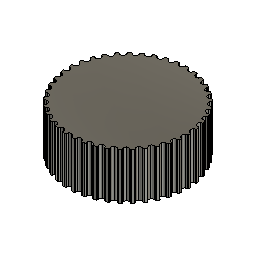
gear_41z (Autodesk Fusion 360 design; units mm, degrees)
Autodesk Fusion 360 part; units mm, degrees
sketch "Sketch1" plane through (0, 0, 0) normal (0, 0, 1) x (1, 0, 0) in component "gt2 pulley"
  circle A0 centre (0, 0) radius 13.0507 construction
  circle A1 centre (0, 0) radius 12.0467 construction
  line L0 (0, 0) -> (0, 13.0507) construction
  line L1 (0, 0) -> (0.999, 13.0124) construction
  line L2 (0, 0) -> (1.4084, 12.9745) construction
  circle A2 centre (0, 0) radius 12.7967 construction
  arc A3 (0.3832, 12.6546) -> (0.4455, 12.3686) centre (1.3809, 12.722) ccw
  circle A4 centre (0, 0) radius 12.6467 construction
  arc A5 (0.2363, 12.7945) -> (0, 12.7967) centre (0, 0) ccw
  arc A6 (0.3832, 12.6546) -> (0.2363, 12.7945) centre (0.2336, 12.6445) ccw
  arc A7 (0.4455, 12.3686) -> (0.9222, 12.0114) centre (0.9647, 12.5647) ccw
  arc A8 (0, 12.7967) -> (-0.2363, 12.7945) centre (0, 0) ccw
  arc A9 (-0.2363, 12.7945) -> (-0.3832, 12.6546) centre (-0.2336, 12.6445) ccw
  arc A10 (-0.4455, 12.3686) -> (-0.3832, 12.6546) centre (-1.3809, 12.722) ccw
  arc A11 (-0.9223, 12.0113) -> (-0.4455, 12.3686) centre (-0.9647, 12.5647) ccw
  arc A12 (0.9222, 12.0114) -> (-0.9222, 12.0114) centre (0, 0) ccw
  point P0 (1.3809, 12.722)
  point P1 (0, 12.7967)
  dimension "d18" = 26.1014
  dimension "d19" = 4.39
  dimension "d22" = 1.004
  dimension "d24" = 0.75
  dimension "d26" = 1
  dimension "d27" = 0.15
  dimension "d28" = 0.15
  dimension "d47" = 0.555
  dimension "d52" = 3.812
  constraint coincident A0.centre A1.centre
  constraint coincident A0 L0.end
  constraint vertical L0
  constraint coincident A0 L1.end
  constraint coincident A0 L2.end
  constraint concentric A1 A2
  constraint coincident A1 A7.end
  constraint coincident L1 A7.end
  constraint coincident A2 P0
  constraint coincident L2 P0
  constraint coincident P0 A3.centre
  constraint coincident A2 P1
  constraint coincident L0 P1
  constraint concentric A2 A4
  constraint coincident P1 A5.end
  constraint coincident A4 A6.centre
  constraint coincident A3.start A6.start
  constraint tangent A3 A6
  constraint tangent A3 A7
  constraint symmetric L0 A7.end A12.end
  constraint symmetric L0 A3.start A9.end
  constraint symmetric L0 A3.end A10.start
  constraint symmetric L0 A3 A10
  constraint symmetric L0 A5.start A8.end
  constraint symmetric L0 P1 A5.end
  constraint symmetric L0 A5 A8
  constraint symmetric L0 A6 A9
  constraint symmetric L0 A7 A11
  constraint coincident A1 A11.start
  constraint tangent A1 A7
  constraint coincident L1 A7.centre
  measures "d18" diameter of A0
  measures "d19" angle of L0 L1
  measures "d22" distance of A0 A1
  measures "d24" distance of A1 A2
  measures "d26" radius of A3
  measures "d27" distance of A2 A4
  measures "d28" radius of A6
  measures "d47" radius of A7
extrude "Extrude1" add sketch "Sketch1" along normal blind 10 makes body 1
pattern_circular "C-Pattern1" count 41 over 360 about axis through (0, 0, 1.75) along (0, 0, 1) of bodies 1 makes body 2 at (-2.5449, 11.7748, 6.6667) makes body 3 at (-4.3125, 11.2483, 6.6667) makes body 4 at (-4.6929, 11.095, 3.3333) makes body 5 at (-7.5054, 9.423, 6.6667) makes body 6 at (-7.8218, 9.162, 3.3333) makes body 7 at (-9.1287, 7.8607, 3.3333) makes body 8 at (-10.2216, 6.3751, 3.3333) makes body 9 at (-11.5601, 3.3893, 6.6667) makes body 10 at (-11.6688, 2.9939, 3.3333) makes body 11 at (-12.044, -0.2565, 6.6667) makes body 12 at (-11.8637, -2.092, 6.6667) makes body 13 at (-11.5885, -3.291, 6.6667) makes body 14 at (-10.6796, -5.5741, 6.6667) makes body 15 at (-9.7035, -7.139, 6.6667) makes body 16 at (-8.9249, -8.0913, 6.6667) makes body 17 at (-7.0973, -9.734, 6.6667) makes body 18 at (-5.5283, -10.7033, 6.6667) makes body 19 at (-5.1608, -10.8853, 3.3333) makes body 20 at (-2.0412, -11.8725, 6.6667) makes body 21 at (-1.6359, -11.9351, 3.3333) makes body 22 at (1.6361, -11.9351, 6.6667) makes body 23 at (2.0414, -11.8725, 3.3333) makes body 24 at (5.1609, -10.8852, 6.6667) makes body 25 at (6.762, -9.9698, 6.6667) makes body 26 at (7.7435, -9.2282, 6.6667) makes body 27 at (9.0615, -7.9381, 6.6667) makes body 28 at (9.7036, -7.1388, 3.3333) makes body 29 at (11.2667, -4.2643, 6.6667) makes body 30 at (11.4053, -3.8783, 3.3333) makes body 31 at (11.8637, -2.0919, 3.3333) makes body 32 at (11.989, 1.1777, 6.6667) makes body 33 at (11.8064, 2.3943, 6.6667) makes body 34 at (11.0749, 4.7402, 6.6667) makes body 35 at (10.5338, 5.8449, 6.6667) makes body 36 at (9.1286, 7.8608, 6.6667) makes body 37 at (7.8216, 9.1622, 6.6667) makes body 38 at (6.3314, 10.2487, 6.6667) makes body 39 at (5.9789, 10.4583, 3.3333) makes body 40 at (4.3123, 11.2484, 3.3333) makes body 41 at (2.5447, 11.7749, 3.3333)
sketch "Sketch2" plane through (0, 0, 10) normal (0, 0, 1) x (-1, 0, 0)
  arc A0 (-10.2965, -7.3668) -> (-10.3186, -7.5685) centre (-10.1977, -7.4797) ccw
  arc A1 (-10.3186, -7.5685) -> (-10.0322, -7.9443) centre (0, 0) ccw
  arc A2 (-10.0322, -7.9443) -> (-9.8318, -7.9763) centre (-9.9145, -7.8512) ccw
  arc A3 (-9.5666, -7.8524) -> (-9.8318, -7.9763) centre (-9.2805, -8.8106) ccw
  arc A4 (-8.9935, -8.015) -> (-9.5666, -7.8524) centre (-9.4078, -8.3842) ccw
  arc A5 (-10.1116, -6.5482) -> (-8.9935, -8.015) centre (0, 0) ccw
  arc A6 (-10.1067, -7.1439) -> (-10.1116, -6.5482) centre (-10.5774, -6.8499) ccw
  arc A7 (-10.2965, -7.3668) -> (-10.1067, -7.1439) centre (-10.9549, -6.6141) ccw
  circle A8 centre (0, 0) radius 12.0467
  constraint coincident A1.centre A5.centre
extrude "Extrude2" add sketch "Sketch2" against normal blind 10 contours A5 A8 bodies 1 2 3 4 5 6 7 8 9 10 11 12 13 14 15 16 17 18 19 20 21 22 23 24 25 26 27 28 29 30 31 32 33 34 35 36 37 38 39 40 41
extrude "Extrude4" [suppressed] in component "gt2 pulley"
pattern_circular "C-Pattern7" [suppressed] in component "gt2 pulley"
extrude "Extrude3" [suppressed] in component "gt2 pulley"
pattern_circular "C-Pattern6" [suppressed] in component "gt2 pulley"
extrude "Extrude2'" [suppressed] in component "gt2 pulley"
pattern_circular "C-Pattern5" [suppressed] in component "gt2 pulley"
extrude "Extrude1'" [suppressed] in component "gt2 pulley"
pattern_circular "C-Pattern4" [suppressed] in component "gt2 pulley"
pattern_circular "C-Pattern3" [suppressed] in component "gt2 pulley"
pattern_circular "C-Pattern2" [suppressed] in component "gt2 pulley"
pattern_circular "C-Pattern1'" [suppressed] in component "gt2 pulley"
copy_body "Body->Comp1" [suppressed] in component "Component"
copy_body "Body->Comp2" [suppressed] in component "Component'"
copy_body "Body->Comp3" [suppressed] in component "Component''"
copy_body "Body->Comp4" [suppressed] in component "Component'''"
copy_body "Body->Comp5" [suppressed] in component "Component''''"
copy_body "Body->Comp6" [suppressed] in component "Component'''''"
copy_body "Body->Comp7" [suppressed] in component "Component''''''"
copy_body "Body->Comp8" [suppressed] in component "Component'''''''"
copy_body "Body->Comp9" [suppressed] in component "Component''''''''"
copy_body "Body->Comp10" [suppressed] in component "Component'''''''''"
copy_body "Body->Comp11" [suppressed] in component "Component''''''''''"
copy_body "Body->Comp12" [suppressed] in component "Component'''''''''''"
copy_body "Body->Comp13" [suppressed] in component "Component''''''''''''"
copy_body "Body->Comp14" [suppressed] in component "Component'''''''''''''"
copy_body "Body->Comp15" [suppressed] in component "Component''''''''''''''"
copy_body "Body->Comp16" [suppressed] in component "Component'''''''''''''''"
copy_body "Body->Comp17" [suppressed] in component "Component''''''''''''''''"
copy_body "Body->Comp18" [suppressed] in component "Component'''''''''''''''''"
copy_body "Body->Comp19" [suppressed] in component "Component''''''''''''''''''"
copy_body "Body->Comp20" [suppressed] in component "Component'''''''''''''''''''"
component "gt2 pulley" placed x (1, 0, 0) y (0, 1, 0) z (0, 0, 1) at (0, 0, 0)
equation "NumTeeth = 41" comment "min 20"
equation "ToothPitch = 2 mm"
equation "PullyDia = NumTeeth * ToothPitch / PI"
equation "ToothAng = ( ( 360 / NumTeeth ) * 1 deg )"
equation "TransOffsetAngle = ToothAng * 0.2"
equation "Sholulder_Radius = 0.15 mm"
equation "Root_Radius = 0.555 mm"
equation "TransRadius = 1 mm"
equation "ToolHeight = 0.75 mm"
equation "PLD = 0.254 mm"
equation "d18 = PullyDia"
equation "d19 = ToothAng / 2"
equation "d22 = PLD + ToolHeight"
equation "d24 = ToolHeight"
equation "d26 = TransRadius"
equation "d27 = Sholulder_Radius"
equation "d31 = NumTeeth"
equation "d33 = NumTeeth"
equation "d35 = NumTeeth"
equation "d37 = NumTeeth"
equation "d41 = NumTeeth"
equation "d45 = NumTeeth"
equation "d47 = Root_Radius"
equation "d50 = NumTeeth"
